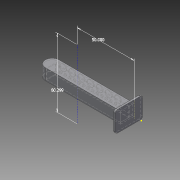
# Autodesk Inventor part: LineArray
Saved by Autodesk Inventor 2015 (Build 190159000, 159)
## iProperties
Created: 2015-02-02
Part Number: LineArray
Material: Generic
Document SubType Name: Modeling
Designer: rubidium
Density: 1 g/cm^3
Appearance: Default
Mass: 42148.7 g
Surface Area: 42208.6 cm^2
Volume: 42148.7 cm^3
Author: rubidium
Autodesk Inventor part; units mm, degrees
ref_plane "YZ Plane" through (0, 0, 0) normal (1, 0, 0) x (0, 1, 0)
ref_plane "XZ Plane" through (0, 0, 0) normal (0, 1, 0) x (-1, 0, 0)
ref_plane "XY Plane" through (0, 0, 0) normal (0, 0, 1) x (1, 0, 0)
sketch "Sketch1" plane through (0, 0, 0) normal (0, 1, 0) x (-1, 0, 0)
  line L0 (1839.667, -285.297) -> (163.267, -285.297)
  line L1 (163.267, -285.297) -> (163.267, -590.097)
  line L2 (163.267, -590.097) -> (1839.667, -590.097)
  arc A0 (1839.667, -590.097) -> (1839.667, -285.297) centre (1839.667, -437.697) ccw
  line L3 (1839.667, -590.097) -> (1839.667, -285.297) construction
  point P0 (0, 0)
  dimension "d0" = 1828.8
  dimension "d2" = 152.4
  dimension "d5" = 304.8
  dimension "d43" = 590.097
  dimension "d59" = 1839.667
  constraints: 8 end point, 2 perpendicular, 2 point on circle, 1 centre point, 1 horizontal, 1 tangent
  measures "d2" radius of A0
  measures "d5" distance of L0.end L1.end
  measures "d43" distance from line of point (0, 0) L2
  measures "d59" distance from line of point (0, 0) L3
extrude "Extrusion1" add sketch "Sketch1" along normal blind 254
shell "Shell1" thickness 17.8562 removed faces 0
sketch "Sketch2" plane through (-163.267, 0, -590.097) normal (0, 0, -1) x (-1, 0, 0)
  circle A0 centre (355.6, 158.75) radius 73.025
  line L0 (0, 0) -> (0, 254) projected
  line L1 (0, 254) -> (1676.4, 254) projected
  circle A1 centre (558.8, 158.75) radius 73.025
  circle A2 centre (762, 158.75) radius 73.025
  circle A3 centre (965.2, 158.75) radius 73.025
  circle A4 centre (1168.4, 158.75) radius 73.025
  circle A5 centre (1371.6, 158.75) radius 73.025
  circle A6 centre (1574.8, 158.75) radius 73.025
  circle A7 centre (304.8, 44.45) radius 25.4
  circle A8 centre (406.4, 44.45) radius 25.4
  circle A9 centre (508, 44.45) radius 25.4
  circle A10 centre (609.6, 44.45) radius 25.4
  circle A11 centre (711.2, 44.45) radius 25.4
  circle A12 centre (812.8, 44.45) radius 25.4
  circle A13 centre (914.4, 44.45) radius 25.4
  circle A14 centre (1016, 44.45) radius 25.4
  circle A15 centre (1117.6, 44.45) radius 25.4
  circle A16 centre (1219.2, 44.45) radius 25.4
  circle A17 centre (1320.8, 44.45) radius 25.4
  circle A18 centre (1422.4, 44.45) radius 25.4
  circle A19 centre (1524, 44.45) radius 25.4
  circle A20 centre (1625.6, 44.45) radius 25.4
  point P0 (-163.267, 0)
  dimension "d11" = 146.05
  dimension "d12" = 355.6
  dimension "d13" = 95.25
  dimension "d19" = 203.2
  dimension "d21" = 304.8
  dimension "d22" = 209.55
  dimension "d23" = 50.8
  dimension "d26" = 101.6
  constraints: 21 centre point, 2 horizontal, 38 other
  measures "d11" diameter of A0
  measures "d12" distance from line of A0.centre L0
  measures "d13" distance from line of L1 A0.centre
  measures "d19" distance of A0.centre A1.centre
  measures "d21" distance from line of L0 A7.centre
  measures "d22" distance from line of L1 A7.centre
  measures "d23" diameter of A7
  measures "d26" distance of A7.centre A8.centre
extrude "Extrusion4" cut sketch "Sketch2" against normal blind 50.8
sketch "Sketch9" plane through (-163.267, 0, -285.297) normal (1, 0, 0) x (0, 0, -1)
  line L0 (406.4, -101.6) -> (-101.6, -101.6)
  line L1 (-152.4, -50.8) -> (-152.4, 304.8)
  line L2 (-101.6, 355.6) -> (406.4, 355.6)
  line L3 (457.2, 304.8) -> (457.2, -50.8)
  line L4 (304.8, 0) -> (0, 0) construction
  line L5 (152.4, 0) -> (152.4, -101.6) construction
  line L6 (304.8, 0) -> (304.8, 254) construction
  line L7 (304.8, 127) -> (457.2, 127) construction
  arc A0 (406.4, -101.6) -> (457.2, -50.8) centre (406.4, -50.8) ccw
  arc A1 (-152.4, -50.8) -> (-101.6, -101.6) centre (-101.6, -50.8) ccw
  arc A2 (-101.6, 355.6) -> (-152.4, 304.8) centre (-101.6, 304.8) ccw
  arc A3 (457.2, 304.8) -> (406.4, 355.6) centre (406.4, 304.8) ccw
  point P0 (-285.297, 0)
  point P1 (457.2, -101.6)
  point P2 (-152.4, -101.6)
  point P3 (457.2, 355.6)
  dimension "d50" = 457.2
  dimension "d51" = 609.6
  dimension "d52" = 50.8
  constraints: 12 end point, 8 point on circle, 8 tangent, 6 point on line, 4 centre point, 4 midpoint, 3 equal radius, 3 perpendicular, 2 parallel, 1 horizontal
  measures "d50" distance of point (457.2, 355.6) point (457.2, -101.6)
  measures "d51" distance of point (457.2, -101.6) point (-152.4, -101.6)
  measures "d52" radius of A0
extrude "Extrusion5" add sketch "Sketch9" along normal blind 37.084
sketch "Sketch10" plane through (-1839.667, 0, -590.097) normal (0, 0, -1) x (-1, 0, 0)
  line L0 (-406.4, 751.6147) -> (-406.4, -779.9775) construction
  line L1 (-1676.4, 304.8) -> (-1676.4, -50.8) construction
  point P0 (-1839.667, 0)
  dimension "d55" = 1531.5921
  dimension "d56" = 1270
  constraints: 2 end point, 1 vertical
  measures "d55" distance of L0.start L0.end
  measures "d56" distance between parallel lines of L1 L0
sketch "Sketch11" plane through (0, 254, 0) normal (0, 1, 0) x (1, 0, 0)
  line L0 (-1839.667, 285.297) -> (-1839.667, 590.097)
  line L1 (-1839.667, 590.097) -> (-1821.125, 590.097)
  line L2 (-163.267, 590.097) -> (-1839.667, 590.097) projected
  arc A0 (-1839.667, 590.097) -> (-1839.667, 285.297) centre (-1839.667, 437.697) ccw projected
  line L3 (-1821.887, 285.297) -> (-1839.667, 285.297)
  line L4 (-1821.887, 285.297) -> (-1821.887, 590.097)
  line L5 (-1821.887, 590.097) -> (-1839.667, 590.097)
  point P0 (0, 0)
  dimension "d58" = 17.78
  constraints: 10 end point, 3 tangent, 2 perpendicular, 2 point on line, 1 parallel, 1 vertical
  measures "d58" distance between parallel lines of L4 L0
extrude "Extrusion6" add sketch "Sketch11" against normal blind 254 contours L0 L1 L4 L3
sketch "Sketch12" plane through (-1821.887, 17.8562, -303.1532) normal (1, 0, 0) x (0, 0, -1)
  line L0 (269.0876, 218.2876) -> (0, 218.2876) projected
  line L1 (198.0438, 218.2876) -> (198.0438, 0)
  line L2 (0, 0) -> (269.0876, 0) projected
  line L3 (198.0438, 0) -> (180.2638, 0)
  line L4 (180.2638, 0) -> (180.2638, 218.2876)
  line L5 (180.2638, 218.2876) -> (198.0438, 218.2876)
  line L6 (286.9438, -17.8562) -> (286.9438, 236.1438) projected
  point P0 (-303.1532, -17.8562)
  dimension "d62" = 17.78
  dimension "d63" = 88.9
  constraints: 8 end point, 4 point on line, 2 perpendicular, 1 vertical
  measures "d62" distance between parallel lines of L4 L1
  measures "d63" distance between parallel lines of L1 L6
extrude "Extrusion7" add sketch "Sketch12" along normal blind 1651
body "Solid1"
